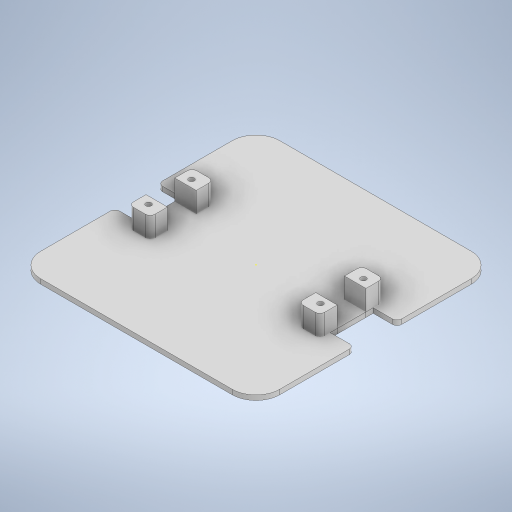
# Autodesk Inventor part: heheheha
Saved by Autodesk Inventor 2023 (Build 270158000, 158)
## iProperties
Created: 2022-12-15
Part Number: heheheha
Material: Ogólny
Document SubType Name: Modeling
Designer: User
Density: 1 g/cm^3
Appearance: Domyślna
Author: User
Autodesk Inventor part; units mm, degrees
ref_plane "YZ Plane" through (0, 0, 0) normal (1, 0, 0) x (0, 1, 0)
ref_plane "XZ Plane" through (0, 0, 0) normal (0, 1, 0) x (-1, 0, 0)
ref_plane "XY Plane" through (0, 0, 0) normal (0, 0, 1) x (1, 0, 0)
sketch "Szkic2" plane through (0, 0, 0) normal (0, 1, 0) x (-1, 0, 0)
  line L0 (50, -50) -> (-50, -50)
  line L1 (50, -50) -> (50, 50)
  line L2 (0, -53.6442) -> (0, 78.3558)
  line L3 (50, 50) -> (-50, 50)
  line L4 (-50, -50) -> (-50, 50)
  line L5 (67.5466, 0) -> (-74.1589, 0)
  line L6 (50, -9) -> (40, -9)
  line L7 (40, -9) -> (40, 9)
  line L8 (40, 9) -> (50, 9)
  line L9 (50, 9) -> (50, -9)
  line L10 (-50, -9) -> (-40, -9)
  line L11 (-40, -9) -> (-40, 9)
  line L12 (-40, 9) -> (-50, 9)
  line L13 (-50, 9) -> (-50, -9)
  line L14 (40, -7.5) -> (31, -7.5)
  line L15 (31, -7.5) -> (31, 7.5)
  line L16 (31, 7.5) -> (40, 7.5)
  line L17 (40, 7.5) -> (40, -7.5)
  line L18 (-40, -7.5) -> (-28.5, -7.5)
  line L19 (-28.5, -7.5) -> (-28.5, 7.5)
  line L20 (-28.5, 7.5) -> (-40, 7.5)
  line L21 (-40, 7.5) -> (-40, -7.5)
  line L22 (31.5, 9) -> (-31.5, 9)
  line L23 (31, 7.5) -> (31, 9)
  line L24 (-28.5, 7.5) -> (-28.5, 9)
  line L25 (31.5, -9) -> (-31.5, -9)
  line L26 (-28.5, -7.5) -> (-28.5, -9)
  line L27 (31, -7.5) -> (31, -9)
  line L28 (40, -11.25) -> (40, -9)
  line L29 (40, 11.25) -> (40, 9)
  line L30 (-40, -11.25) -> (-40, -9)
  line L31 (-40, 11.25) -> (-40, 9)
  circle A0 centre (35.95, -9) radius 1.15
  line L32 (40, -9) -> (40, -7.5)
  line L33 (-40, -9) -> (-40, -7.5)
  line L34 (40, 9) -> (40, 7.5)
  line L35 (-40, 9) -> (-40, 7.5)
  line L36 (40, -9) -> (40, -9)
  line L37 (40, 9) -> (40, 9)
  line L38 (-40, -9) -> (-40, -9)
  line L39 (-40, 9) -> (-40, 9)
  circle A1 centre (35.95, 9) radius 1.15
  circle A2 centre (-35.95, -9) radius 1.15
  circle A3 centre (-35.95, 9) radius 1.15
  line L40 (37.1, -9) -> (37.1, -7.5)
  line L41 (34.8, -9) -> (34.8, -7.5)
  line L42 (40, -14.25) -> (40, -13.75)
  line L43 (37.1, 9) -> (37.1, 7.5)
  line L44 (34.8, 9) -> (34.8, 7.5)
  line L45 (31, 5.5681) -> (31, 11.25)
  line L46 (33, 13.25) -> (38, 13.25)
  line L47 (40, 14.25) -> (40, 13.75)
  circle A4 centre (-35.95, -9) radius 1.15
  line L48 (-37.1, -9) -> (-37.1, -7.5)
  line L49 (-34.8, -9) -> (-34.8, -7.5)
  circle A5 centre (-35.95, 9) radius 1.15
  line L50 (-37.1, 9) -> (-37.1, 7.5)
  line L51 (-34.8, 9) -> (-34.8, 7.5)
  line L52 (-40, -14.25) -> (-40, -13.75)
  line L53 (-31, 9) -> (-31, 11.25)
  line L54 (-40, 14.25) -> (-40, 14.75)
  line L55 (50, -50) -> (50, 50)
  line L56 (50, -50) -> (-50, -50)
  line L57 (50, -9) -> (40, -9)
  line L58 (40, 9) -> (50, 9)
  line L59 (40, 7.5) -> (40, -7.5)
  line L60 (50, -50) -> (-50, -50)
  line L61 (-40, 0) -> (-9.8, 0)
  line L62 (-9.7869, 9) -> (-9.7869, -9)
  line L63 (9.7869, 9) -> (9.7869, -9)
  line L64 (40, -6) -> (31, -6)
  line L65 (40, 6) -> (31, 6)
  line L66 (40, -13.75) -> (40, -9)
  line L67 (31, -5.5681) -> (31, -11.25)
  line L68 (33, -13.25) -> (38, -13.25)
  line L69 (-40, -7.5) -> (-31, -7.5)
  line L70 (-31, 7.5) -> (-40, 7.5)
  circle A6 centre (-35.95, -9) radius 1.15
  circle A7 centre (-35.95, 9) radius 1.15
  line L71 (-37.1, -9) -> (-37.1, -7.5)
  line L72 (-34.8, -9) -> (-34.8, -7.5)
  line L73 (-37.1, 9) -> (-37.1, 7.5)
  line L74 (-34.8, 9) -> (-34.8, 7.5)
  line L75 (-31, 5.5681) -> (-31, 13.25)
  line L76 (-33, 13.25) -> (-38, 13.25)
  line L77 (-40, -6) -> (-31, -6)
  line L78 (-33, -13.25) -> (-38, -13.25)
  line L79 (-31, -5.5681) -> (-31, -11.25)
  arc A8 (38, -13.25) -> (40, -11.25) centre (38, -11.25) ccw
  arc A9 (31, -11.25) -> (33, -13.25) centre (33, -11.25) ccw
  arc A10 (40, 11.25) -> (38, 13.25) centre (38, 11.25) ccw
  arc A11 (33, 13.25) -> (31, 11.25) centre (33, 11.25) ccw
  arc A12 (-31, 11.25) -> (-33, 13.25) centre (-33, 11.25) ccw
  arc A13 (-38, 13.25) -> (-40, 11.25) centre (-38, 11.25) ccw
  arc A14 (-40, -11.25) -> (-38, -13.25) centre (-38, -11.25) ccw
  arc A15 (-33, -13.25) -> (-31, -11.25) centre (-33, -11.25) ccw
  line L80 (-40, 6) -> (-31, 6)
  point P0 (0, 0)
  point P1 (-50, 9)
  point P2 (-34.25, -7.5)
  point P3 (27.1, -10.7133)
  point P4 (31.5, -9)
  point P5 (31.5, -9)
  point P6 (-31.5, 9)
  point P7 (-31.5, 9)
  point P8 (27.1, 10.7133)
  point P9 (40, 7.5)
  point P10 (31, 13.25)
  point P11 (40.0775, 13.25)
  point P12 (-31, -9)
  point P13 (-31, -14.25)
  point P14 (-31, 15.2922)
  point P15 (-34.8, 9)
  point P16 (-37.1, 9)
  point P17 (-37.1, 7.5)
  point P18 (-34.8, 7.5)
  point P19 (-31, 9)
  point P20 (-37.1, -9)
  point P21 (-34.8, -9)
  point P22 (-34.8, -7.5)
  point P23 (-37.1, -7.5)
  point P24 (37.1, 9)
  point P25 (34.8, 9)
  point P26 (34.8, 7.5)
  point P27 (37.1, 7.5)
  point P28 (31, 9)
  point P29 (-50, 0)
  point P30 (31, -13.25)
  point P31 (40.0775, -13.25)
  point P32 (-40.0775, 13.25)
  point P33 (-31, -13.25)
  point P34 (-40.0775, -13.25)
  dimension "d30" = 100
  dimension "d31" = 132
  dimension "d32" = 18
  dimension "d33" = 10
  dimension "d38" = 9
  dimension "d39" = 15
  dimension "d40" = 15
  dimension "d41" = 11.5
  dimension "d42" = 10
  dimension "d44" = 15
  dimension "d47" = 0
  dimension "d50" = 2.3
  dimension "d59" = 2.9
  dimension "d62" = 0.5
  dimension "d68" = 100
  dimension "d69" = 50
  dimension "d70" = 30.2
  dimension "d71" = 1.5
  dimension "d73" = 5.75
  dimension "d74" = 2
  constraints: 158 end point, 51 symmetric about line, 32 point on line, 22 point on circle, 18 tangent, 16 centre point, 14 horizontal, 12 vertical, 9 parallel, 8 perpendicular, 7 equal radius, 7 midpoint, 1 collinear, 68 other
  measures "d30" distance of L0.start L0.end
  measures "d31" distance of L2.start L2.end
  measures "d32" distance of L6.end L7.end
  measures "d33" distance of L6.start L6.end
  measures "d38" distance of L14.start L14.end
  measures "d39" distance of L14.end L15.end
  measures "d40" distance of L20.end L18.start
  measures "d41" distance of L18.start L18.end
  measures "d42" distance of L10.start L10.end
  measures "d44" distance from line of L20 point (-34.25, -7.5)
  measures "d47" distance of L6.end L32.start
  measures "d50" diameter of A0
  measures "d59" distance of L14.start L40.end
  measures "d62" distance of L52.end L52.start
  measures "d68" distance of L0.end L3.end
  measures "d69" distance of point (-50, 0) L3.end
  measures "d70" distance of L61.start L61.end
  measures "d71" distance between parallel lines of L64 L14
  measures "d73" distance between parallel lines of L68 L14
  measures "d74" radius of A8
extrude "Wyciągnięcie proste3" add sketch "Szkic2" along normal blind 10.5 contours L28 A8 L68 A9 L67 L27 L14 L41 A0 L40 L7 | L14 L15 L64 L7 | L11 L18 L48 A2 L49 L79 A15 L78 A14 L30 | L7 L16 L43 A1 L44 L23 L45 A11 L46 A10 L29 | L65 L15 L16 L7 | L40 A0 L41 L14 | L11 L77 L79 L18 | L31 A13 L76 A12 L53 L75 L20 L51 A3 L50 L11 | L11 L20 L75 L80 | L18 L49 A2 L48 | L16 L44 A1 L43 | L50 A3 L51 L20
extrude "Wyciągnięcie proste4" add sketch "Szkic2" along normal blind 2 separate body contours L0 L2 L25 L67 A9 L68 A8 L28 L6 L1 | L0 L4 L10 L30 A14 L78 A15 L79 L25 L2 | L25 L62 L5 L2 | L2 L5 L63 L25 | L28 A8 L68 A9 L67 L27 L14 L41 A0 L40 L7 | L5 L62 L22 L2 | L2 L22 L63 L5 | L63 L5 L15 L27 L25 | L25 L26 L19 L5 L62 | L8 L29 A10 L46 A11 L45 L22 L2 L3 L1 | L7 L64 L15 L5 | L5 L15 L65 L7 | L14 L15 L64 L7 | L11 L18 L48 A2 L49 L79 A15 L78 A14 L30 | L22 L53 A12 L76 A13 L31 L12 L4 L3 L2 | L63 L22 L23 L15 L5 | L5 L19 L24 L22 L62 | L25 L79 L18 L26 | L7 L16 L43 A1 L44 L23 L45 A11 L46 A10 L29 | L65 L15 L16 L7 | L40 A0 L41 L14 | L11 L80 L75 L20 L19 L5 | L5 L19 L18 L79 L77 L11 | L11 L77 L79 L18 | A0 | L31 A13 L76 A12 L53 L75 L20 L51 A3 L50 L11 | L11 L20 L75 L80 | L18 L49 A2 L48 | L24 L20 L75 L22 | L16 L44 A1 L43 | A2 | A1 | L50 A3 L51 L20 | A3
fillet "Zaokrąglenie4" radius 10 4 edges at (-50, 1, -50) (-50, 1, 50) (50, 1, 50) (50, 1, -50)
fillet "Zaokrąglenie5" radius 2 4 edges at (50, 1, 9) (50, 1, -9) (-50, 1, 9) (-50, 1, -9)
sketch "Szkic3" plane through (0, 2, 0) normal (0, 1, 0) x (1, 0, 0)
  point P0 (0, 0)
